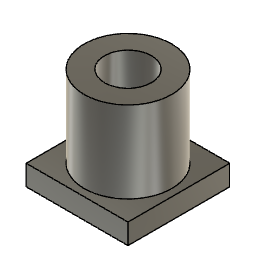
Halterung Gewindeeinsatz v1 (Autodesk Fusion 360 design; units mm, degrees)
Autodesk Fusion 360 part; units mm, degrees
sketch "Skizze1" plane through (0, 0, 0) normal (0, 0, 1) x (1, 0, 0)
  line L0 (-4, 4) -> (4, 4)
  line L1 (4, 4) -> (4, -4)
  line L2 (4, -4) -> (-4, -4)
  line L3 (-4, -4) -> (-4, 4)
  line L4 (-4, 4) -> (4, -4) construction
  line L5 (4, 4) -> (-4, -4) construction
  dimension "d1" = 8
  dimension "d2" = 8
  constraint horizontal L0
  constraint perpendicular L0 L1
  constraint parallel L0 L2
  constraint parallel L1 L3
  constraint coincident L4 origin
  constraint coincident L5 origin
  measures "d1" distance of L1.end L2.end
  measures "d2" distance of L0.end L1.end
extrude "Extrusion1" add sketch "Skizze1" along normal blind 2
sketch "Skizze2" plane through (0, 0, 2) normal (0, 0, 1) x (-1, 0, 0)
  line L0 (4, 4) -> (-4, 4)
  line L1 (-4, 4) -> (-4, -4)
  line L2 (-4, -4) -> (4, -4)
  line L3 (4, -4) -> (4, 4)
  circle A0 centre (0, 0) radius 2.3
  circle A1 centre (0, 0) radius 3.3
  dimension "d5" = 4.6
  dimension "d6" = 6.6
  constraint coincident A0.centre A1.centre
  measures "d5" diameter of A0
  measures "d6" diameter of A1
extrude "Extrusion2" add sketch "Skizze2" along normal blind 8 contours A1
extrude "Extrusion3" add 1 faces at (0.6334, 0.4319, 2) along direction (0, 0, 1) blind 2
extrude "Extrusion4" add 1 faces at (1.3333, -4, 0.6667) along direction (0, -1, 0) blind 1
extrude "Extrusion5" add 1 faces at (4, 1, 0.6667) along direction (1, 0, 0) blind 1
extrude "Extrusion6" add 1 faces at (2, 4, 1.3333) along direction (0, 1, 0) blind 1
extrude "Extrusion7" add 1 faces at (-4, 1.6667, 0.6667) along direction (-1, 0, 0) blind 1
move_face "Flächen versetzen1" offset 1 1 faces at (-3.2959, 0.1645, 7.3333)
